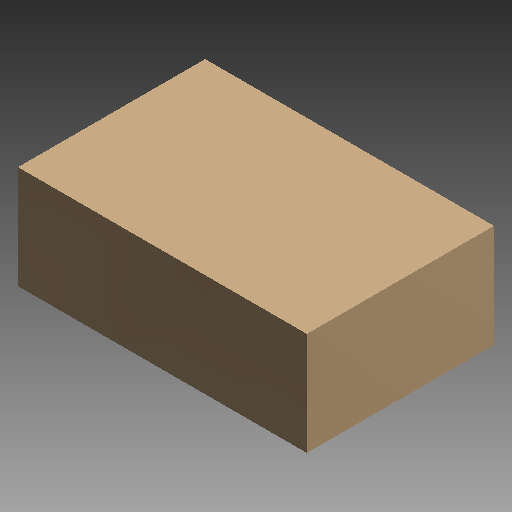
# Autodesk Inventor part: 3557-2
Saved by Autodesk Inventor 2018.2 (Build 222227000, 227)
## iProperties
Part Number: 3557-2
Material: Generic
Document SubType Name: Modeling
Designer: autocad
Appearance: 3557, 3557-2
Author: autocad
Autodesk Inventor part; units mm, degrees
ref_plane "YZ Plane" through (0, 0, 0) normal (1, 0, 0) x (0, 1, 0)
ref_plane "XZ Plane" through (0, 0, 0) normal (0, 1, 0) x (-1, 0, 0)
ref_plane "XY Plane" through (0, 0, 0) normal (0, 0, 1) x (1, 0, 0)
sketch "3557, 3557-2_76" plane through (0, 0, 0) normal (0, 0, 1) x (1, 0, 0)
  line L0 (-9.9695, -3.556) -> (-9.9695, 3.556)
  line L1 (-9.9695, 3.556) -> (9.9695, 3.556)
  line L2 (9.9695, 3.556) -> (9.9695, -3.556)
  line L3 (9.9695, -3.556) -> (-9.9695, -3.556)
  constraints: 8 end point
extrude "Extrusion1" add sketch "3557, 3557-2_76" along normal blind 12.92
body "Solid1"
